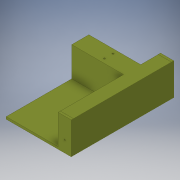
# Autodesk Inventor part: CPLRightThree
Saved by Autodesk Inventor 2019 (Build 230136000, 136)
## iProperties
Created: 2019-01-04
Part Number: CPLRightThree
Material: Generic
Document SubType Name: Modeling
Designer: james
Density: 1 g/cm^3
Appearance: Default(2)
Author: james
Autodesk Inventor part; units mm, degrees
ref_plane "YZ Plane" through (0, 0, 0) normal (1, 0, 0) x (0, 1, 0)
ref_plane "XZ Plane" through (0, 0, 0) normal (0, 1, 0) x (-1, 0, 0)
ref_plane "XY Plane" through (0, 0, 0) normal (0, 0, 1) x (1, 0, 0)
sketch "Sketch51" plane through (0, 0, 0) normal (0, 1, 0) x (-1, 0, 0)
  line L0 (1.3484, 37.0338) -> (-3.7316, 37.0338)
  line L1 (-3.7316, 37.0338) -> (-3.7316, -191.5662)
  line L2 (-3.7316, -191.5662) -> (1.3484, -191.5662)
  line L3 (1.3484, -191.5662) -> (1.3484, 37.0338)
  point P0 (0, 0)
  dimension "d172" = 5.08
  dimension "d173" = 228.6
  constraints: 8 end point, 2 parallel, 1 horizontal, 1 perpendicular
  measures "d172" distance of L0.start L0.end
  measures "d173" distance of L2.end L0.start
extrude "Extrusion37" add sketch "Sketch51" along normal blind 71.12
sketch "Sketch52" plane through (-1.3484, 0, 37.0338) normal (0, 0, 1) x (1, 0, 0)
  line L0 (5.08, 0) -> (5.08, 71.12) projected
  line L1 (5.08, 71.12) -> (-24.13, 71.12)
  line L2 (-24.13, 71.12) -> (-24.13, 66.04)
  line L3 (-24.13, 66.04) -> (5.08, 66.04)
  line L4 (5.08, 66.04) -> (5.08, 71.12)
  point P0 (1.3484, 0)
  dimension "d176" = 5.08
  dimension "d177" = 29.21
  constraints: 8 end point, 2 parallel, 1 horizontal, 1 perpendicular
  measures "d176" distance of L1.end L2.end
  measures "d177" distance of L0.end L1.end
extrude "Extrusion38" add sketch "Sketch52" against normal blind 228.6
sketch "Sketch54" plane through (0, 0, 0) normal (0, -1, 0) x (1, 0, 0)
  line L0 (-20.3984, 37.0338) -> (-141.0484, 37.0338)
  line L1 (-141.0484, 37.0338) -> (-141.0484, -191.5662)
  line L2 (-141.0484, -191.5662) -> (-20.3984, -191.5662)
  line L3 (-20.3984, -191.5662) -> (-20.3984, 37.0338)
  line L4 (-25.4784, 37.0338) -> (-1.3484, 37.0338) projected
  line L5 (-1.3484, -191.5662) -> (-25.4784, -191.5662) projected
  line L6 (-1.3484, -191.5662) -> (-1.3484, 37.0338) projected
  point P0 (0, 0)
  dimension "d180" = 0
  dimension "d181" = 0
  dimension "d182" = 19.05
  dimension "d183" = 120.65
  constraints: 8 end point, 2 parallel, 1 horizontal, 1 perpendicular
  measures "d180" distance between parallel lines of L4 L0
  measures "d181" distance between parallel lines of L5 L2
  measures "d182" distance between parallel lines of L3 L6
  measures "d183" distance of L0.start L0.end
extrude "Extrusion39" add sketch "Sketch54" against normal blind 5.08 contours L3 L2 L1 L0
sketch "Sketch55" plane through (-1.3484, 0, 37.0338) normal (0, 0, 1) x (1, 0, 0)
  line L0 (-139.7, 5.08) -> (-19.05, 5.08) projected
  line L1 (-24.13, 66.04) -> (-24.13, 71.12) projected
  line L2 (-19.05, 5.08) -> (-24.13, 5.08)
  line L3 (-24.13, 5.08) -> (-24.13, 71.12)
  line L4 (-24.13, 71.12) -> (-19.05, 71.12)
  line L5 (-19.05, 71.12) -> (-19.05, 5.08)
  point P0 (1.3484, 0)
  constraints: 8 end point, 2 parallel, 1 horizontal, 1 perpendicular
extrude "Extrusion40" add sketch "Sketch55" against normal blind 228.6
sketch "Sketch56" plane through (3.7316, 0, 37.0338) normal (0, 0, 1) x (1, 0, 0)
  line L0 (-29.4089, 71.1531) -> (0, 71.1531)
  line L1 (0, 71.1531) -> (0, 0)
  line L2 (0, 0) -> (-29.4089, 0)
  line L3 (-29.4089, 0) -> (-29.4089, 71.1531)
  point P0 (-3.7316, 0)
  constraints: 8 end point, 2 parallel, 1 horizontal, 1 perpendicular
extrude "Extrusion41" add sketch "Sketch56" against normal blind 5.08
sketch "Sketch57" plane through (3.7316, 0, -191.5662) normal (0, 0, -1) x (-1, 0, 0)
  line L0 (29.4089, 5.08) -> (29.4089, 71.1531) projected
  line L1 (29.4089, 71.1531) -> (0, 71.1531)
  line L2 (0, 71.1531) -> (0, 0)
  line L3 (0, 0) -> (29.4089, 0)
  line L4 (29.4089, 0) -> (29.4089, 71.1531)
  point P0 (3.7316, 0)
  constraints: 8 end point, 2 parallel, 1 horizontal, 1 perpendicular
extrude "Extrusion42" add sketch "Sketch57" against normal blind 5.08
sketch "Sketch58" plane through (0, 71.12, 0) normal (0, 1, 0) x (1, 0, 0)
  line L0 (-25.4784, -31.9538) -> (-25.4784, 186.4862) projected
  line L1 (-141.0484, 191.5662) -> (-141.0484, -37.0338) projected
  line L2 (-25.4784, 109.0162) -> (-141.0484, 109.0162)
  line L3 (-141.0484, 109.0162) -> (-141.0484, 147.1162)
  line L4 (-141.0484, 147.1162) -> (-25.4784, 147.1162)
  line L5 (-25.4784, 147.1162) -> (-25.4784, 109.0162)
  line L6 (-25.6773, 191.5662) -> (-141.0484, 191.5662) projected
  point P0 (0, 0)
  dimension "d192" = 38.1
  dimension "d193" = 44.45
  constraints: 8 end point, 2 parallel, 2 point on line, 1 horizontal, 1 perpendicular
  measures "d192" distance between parallel lines of L2 L4
  measures "d193" distance between parallel lines of L6 L4
extrude "Extrusion43" add sketch "Sketch58" against normal blind 5.08
sketch "Sketch59" plane through (-141.0484, 71.12, -147.1162) normal (-1, 0, 0) x (0, 0, 1)
  line L0 (0, 0) -> (0, -5.08) projected
  line L1 (184.15, -71.12) -> (-44.45, -71.12) projected
  line L2 (0, 0) -> (5.08, 0)
  line L3 (5.08, 0) -> (5.08, -71.12)
  line L4 (5.08, -71.12) -> (0, -71.12)
  line L5 (0, -71.12) -> (0, 0)
  line L6 (38.1, 0) -> (38.1, -5.08) projected
  line L7 (38.1, 0) -> (33.02, 0)
  line L8 (33.02, 0) -> (33.02, -71.12)
  line L9 (33.02, -71.12) -> (38.1, -71.12)
  line L10 (38.1, -71.12) -> (38.1, 0)
  point P0 (147.1162, -71.12)
  dimension "d196" = 5.08
  dimension "d197" = 5.08
  constraints: 16 end point, 4 parallel, 2 horizontal, 2 perpendicular, 2 point on line
  measures "d196" distance between parallel lines of L3 L5
  measures "d197" distance between parallel lines of L10 L8
extrude "Extrusion44" add sketch "Sketch59" against normal blind 120.65
sketch "Sketch60" plane through (-141.0484, 0, -191.5662) normal (-1, 0, 0) x (0, 0, 1)
  line L0 (49.53, 5.08) -> (77.47, 5.08) projected
  line L1 (5.08, 0) -> (223.52, 0) projected
  line L2 (49.53, 5.08) -> (77.4104, 5.08)
  line L3 (77.4104, 5.08) -> (77.4104, 0)
  line L4 (77.4104, 0) -> (49.53, 0)
  line L5 (49.53, 0) -> (49.53, 5.08)
  point P0 (191.5662, 0)
  constraints: 8 end point, 2 parallel, 1 horizontal, 1 perpendicular, 1 point on line
extrude "Extrusion45" cut sketch "Sketch60" against normal blind 120.65
sketch "Sketch61" plane through (-25.4784, 66.04, -142.0362) normal (-1, 0, 0) x (0, 0, 1)
  line L0 (0, -66.04) -> (0, 0) projected
  line L1 (27.94, 0) -> (27.94, -60.96) projected
  line L2 (27.94, 0) -> (0, 0) projected
  line L3 (-44.45, -66.04) -> (173.99, -66.04) projected
  line L4 (0, 0) -> (27.6512, 0)
  line L5 (27.6512, 0) -> (27.6512, -66.04)
  line L6 (27.6512, -66.04) -> (0, -66.04)
  line L7 (0, -66.04) -> (0, 0)
  point P0 (142.0362, -66.04)
  constraints: 8 end point, 2 parallel, 1 horizontal, 1 perpendicular, 1 point on line
extrude "Extrusion46" cut sketch "Sketch61" against normal blind 5.08
sketch "Sketch62" plane through (-141.0484, 5.08, -109.0162) normal (-1, 0, 0) x (0, 0, 1)
  line L0 (-33.02, -5.08) -> (-82.55, -5.08) projected
  line L1 (-38.1, 66.04) -> (-38.1, 0) projected
  line L2 (0, 66.04) -> (0, 0) projected
  line L3 (-5.1396, 0) -> (-5.1396, -5.08) projected
  line L4 (146.05, -5.08) -> (-5.1396, -5.08) projected
  line L5 (146.05, -5.08) -> (146.05, 0) projected
  line L6 (0, 0) -> (146.05, 0) projected
  line L7 (0, 66.04) -> (0, 0) projected
  line L8 (0, 66.04) -> (-38.1, 66.04) projected
  line L9 (-38.1, 66.04) -> (-38.1, 0) projected
  line L10 (-82.55, 0) -> (-38.1, 0) projected
  line L11 (-82.55, -5.08) -> (-82.55, 0) projected
  line L12 (-33.02, -5.08) -> (-82.55, -5.08) projected
  line L13 (-33.02, -5.08) -> (-33.02, 60.96) projected
  line L14 (-5.08, 60.96) -> (-33.02, 60.96) projected
  line L15 (-5.08, 60.96) -> (-5.08, 0) projected
  line L16 (0, 66.04) -> (-34.1859, 66.04)
  line L17 (-34.1859, 66.04) -> (-34.1859, -5.08)
  line L18 (-34.1859, -5.08) -> (0, -5.08)
  line L19 (0, -5.08) -> (0, 66.04)
  line L20 (-5.1396, 0) -> (-5.08, 0) projected
  point P0 (109.0162, -5.08)
  constraints: 8 end point, 2 parallel, 1 horizontal, 1 perpendicular, 1 point on line
extrude "Extrusion47" add sketch "Sketch62" against normal blind 5.08 contours L0 L17 L8 L2 L19 L4 L3 L20 L15 L14 L13 | L13 L14 L15 L20 L3 L18
sketch "Sketch63" plane through (3.7316, 0, -191.5662) normal (0, 0, -1) x (-1, 0, 0)
  line L0 (0, 0) -> (144.78, 0) projected
  line L1 (29.4089, 5.08) -> (29.4089, 71.1531) projected
  point P0 (3.7316, 0)
  point P1 (14.1689, 25.4)
  dimension "d206" = 25.4
  dimension "d207" = 15.24
  measures "d206" distance from line of L0 point (14.169, 25.4)
  measures "d207" distance from line of L1 point (14.169, 25.4)
hole "Hole8" at (-10.4373, 25.4, -191.5662) direction (0, 0, 1) diameter 3.302 end through all
sketch "Sketch64" plane through (-141.0484, 0, -191.5662) normal (-1, 0, 0) x (0, 0, 1)
  line L0 (228.6, 0) -> (0, 0) projected
  line L1 (44.45, 71.12) -> (44.45, 5.08) projected
  point P0 (191.5662, 0)
  point P1 (63.5, 25.4)
  dimension "d215" = 25.4
  dimension "d216" = 19.05
  measures "d215" distance from line of L0 point (63.5, 25.4)
  measures "d216" distance from line of point (63.5, 25.4) L1
hole "Hole9" at (-141.0484, 25.4, -128.0662) direction (1, 0, 0) diameter 3.302 depth 25.4 tip angle 118.188
sketch "Sketch66" plane through (0, 71.12, 0) normal (0, 1, 0) x (1, 0, 0)
  line L0 (-141.0484, 109.0162) -> (-141.0484, 147.1162) projected
  line L1 (-25.4784, 109.0162) -> (-141.0484, 109.0162) projected
  line L2 (-141.0484, 147.1162) -> (-25.4784, 147.1162) projected
  point P0 (0, 0)
  point P1 (-77.5484, 137.5912)
  point P2 (-77.5484, 118.5412)
  dimension "d224" = 0
  dimension "d225" = 63.5
  dimension "d226" = 9.525
  dimension "d227" = 9.525
  measures "d224" horizontal distance of point (-77.548, 118.541) point (-77.548, 137.591)
  measures "d225" distance from line of L0 point (-77.548, 118.541)
  measures "d226" distance from line of L1 point (-77.548, 118.541)
  measures "d227" distance from line of L2 point (-77.548, 137.591)
hole "Hole10" at (-77.5484, 71.12, -137.5912) at (-77.5484, 71.12, -118.5412) direction (0, -1, 0) diameter 3.81 depth 25.4 tip angle 118.188
equation "\"d172\" = WallWidth"
equation "\"d173\" = PartLength"
equation "\"d174\" = CPDeckHeight"
equation "\"d176\" = WallWidth"
equation "\"d177\" = 2 * WallWidth + ControlPlateShelfLength"
equation "\"d178\" = PartLength"
equation "\"d182\" = ControlPlateShelfLength"
equation "\"d183\" = CPDWidthHole"
equation "\"d184\" = WallWidth"
equation "\"d186\" = PartLength"
equation "\"d188\" = WallWidth"
equation "\"d190\" = WallWidth"
equation "\"d194\" = WallWidth"
equation "\"d196\" = WallWidth"
equation "\"d197\" = WallWidth"
equation "\"d202\" = WallWidth"
equation "\"d204\" = WallWidth"
equation "\"DSLength\" = 1371.6"
equation "\"DSWidth\" = 304.8"
equation "\"DCDeckHeight\" = 76.2"
equation "\"WallWidth\" = 5.08"
equation "\"EdgeAngle\" = 10deg"
equation "\"LengthCuts\" = 152.4"
equation "\"WidthCuts\" = 50.8"
equation "\"PartLength\" = 228.6"
equation "\"PartWidth\" = 152.4"
equation "\"BoltHoldDiam\" = 6.35"
equation "\"ControlPlateLength\" = 228.6"
equation "\"ControlPlateWidth\" = 228.6"
equation "\"ControlPlateShelfLength\" = 19.05"
equation "\"ControlHoleLength\" = 190.5"
equation "\"ControlHoleWidth\" = 190.5"
equation "\"ControlHoleFromSide\" = 63.5"
equation "\"ControlHoleBoltHoleMid\" = 9.525"
equation "\"CPDeckHeight\" = 71.12"
equation "\"CPFromSide\" = 63.5"
equation "\"CPFromBack\" = 63.5"
equation "\"DU1CHWidth\" = 69.85"
equation "\"DU1CHLength\" = 146.05"
equation "\"ControlPlateScrewLength\" = 76.2"
equation "\"DSBackHeight\" = 127"
equation "\"BackShelf\" = 25.4"
equation "\"MainAngle\" = 168.22deg"
equation "\"CPDWidthHole\" = 120.65"
equation "\"CPDLengthHole\" = 146.05"
equation "\"DownBackHeight\" = 130.7084"
body "Solid2"
